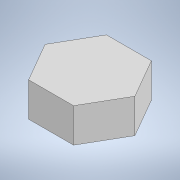
# Autodesk Inventor part: Wheel side stand nut
Saved by Autodesk Inventor 2021 (Build 250183000, 183)
## iProperties
Created: 2021-07-01
Part Number: Wheel side stand nut
Material: Generic
Document SubType Name: Modeling
Designer: Rupali B
Density: 1 g/cm^3
Appearance: Default
Author: Rupali B
Autodesk Inventor part; units mm, degrees
ref_plane "YZ Plane" through (0, 0, 0) normal (1, 0, 0) x (0, 1, 0)
ref_plane "XZ Plane" through (0, 0, 0) normal (0, 1, 0) x (-1, 0, 0)
ref_plane "XY Plane" through (0, 0, 0) normal (0, 0, 1) x (1, 0, 0)
sketch "Sketch1" plane through (0, 0, 0) normal (0, 1, 0) x (-1, 0, 0)
  line L0 (-9.9441, 7.0739) -> (9.9441, 7.0739)
  line L1 (9.9441, 7.0739) -> (9.9441, -7.0739)
  line L2 (9.9441, -7.0739) -> (-9.9441, -7.0739)
  line L3 (-9.9441, -7.0739) -> (-9.9441, 7.0739)
  line L4 (-9.9441, 7.0739) -> (9.9441, -7.0739) construction
  line L5 (9.9441, 7.0739) -> (-9.9441, -7.0739) construction
  line L6 (5.2211, 0) -> (2.6105, -4.5216)
  line L7 (2.6105, -4.5216) -> (-2.6105, -4.5216)
  line L8 (-2.6105, -4.5216) -> (-5.2211, 0)
  line L9 (-5.2211, 0) -> (-2.6105, 4.5216)
  line L10 (-2.6105, 4.5216) -> (2.6105, 4.5216)
  line L11 (2.6105, 4.5216) -> (5.2211, 0)
  point P0 (0, 0)
  point P1 (0, 0)
  dimension "d0" = 19.8882
  dimension "d1" = 14.1478
  constraints: 24 end point, 2 midpoint, 2 parallel, 1 coincident, 1 horizontal, 1 perpendicular, 13 other
  measures "d0" distance of L1.end L2.end
  measures "d1" distance of L0.end L1.end
extrude "Extrusion1" add sketch "Sketch1" along normal blind 3.9688 contours L6 L7 L8 L9 L10 L11
body "Solid1"
